Autodesk Fusion 360 part; units mm, degrees
note: some values were not read from the file. Set by a fixed rule: the direction of a hole.
(part 6 of 10)
  line L4790 (55.322, 32.9023) -> (55.808, 32.999)
  line L4791 (58.348, 32.999) -> (58.834, 32.9023)
  line L4792 (59.246, 32.627) -> (59.5213, 32.215)
  line L4793 (58.348, 30.459) -> (55.808, 30.459)
  line L4794 (55.808, 32.999) -> (58.348, 32.999)
  line L4795 (59.5213, 31.243) -> (59.246, 30.831)
  line L4796 (55.808, 30.459) -> (55.322, 30.5557)
  line L4797 (58.834, 32.9023) -> (59.246, 32.627)
  line L4798 (59.618, 31.729) -> (59.5213, 31.243)
  line L4799 (67.61, 55.627) -> (68.022, 55.9023)
  line L4800 (71.048, 55.999) -> (71.534, 55.9023)
  line L4801 (67.3347, 54.243) -> (67.238, 54.729)
  line L4802 (67.61, 53.831) -> (67.3347, 54.243)
  line L4803 (72.2213, 54.243) -> (71.946, 53.831)
  line L4804 (68.508, 53.459) -> (68.022, 53.5557)
  line L4805 (71.534, 53.5557) -> (71.048, 53.459)
  line L4806 (68.022, 53.5557) -> (67.61, 53.831)
  line L4807 (71.946, 53.831) -> (71.534, 53.5557)
  line L4808 (68.508, 55.999) -> (71.048, 55.999)
  line L4809 (72.2213, 55.215) -> (72.318, 54.729)
  line L4810 (68.022, 55.9023) -> (68.508, 55.999)
  line L4811 (71.946, 55.627) -> (72.2213, 55.215)
  line L4812 (71.048, 53.459) -> (68.508, 53.459)
  line L4813 (71.534, 55.9023) -> (71.946, 55.627)
  line L4814 (72.318, 54.729) -> (72.2213, 54.243)
  line L4815 (67.238, 54.729) -> (67.3347, 55.215)
  line L4816 (67.3347, 55.215) -> (67.61, 55.627)
  line L4817 (67.238, 31.729) -> (67.3347, 32.215)
  line L4818 (67.61, 30.831) -> (67.3347, 31.243)
  line L4819 (68.508, 30.459) -> (68.022, 30.5557)
  line L4820 (68.022, 30.5557) -> (67.61, 30.831)
  line L4821 (72.318, 31.729) -> (72.2213, 31.243)
  line L4822 (67.61, 32.627) -> (68.022, 32.9023)
  line L4823 (71.048, 32.999) -> (71.534, 32.9023)
  line L4824 (67.3347, 32.215) -> (67.61, 32.627)
  line L4825 (71.534, 30.5557) -> (71.048, 30.459)
  line L4826 (67.3347, 31.243) -> (67.238, 31.729)
  line L4827 (68.022, 32.9023) -> (68.508, 32.999)
  line L4828 (71.534, 32.9023) -> (71.946, 32.627)
  line L4829 (72.2213, 31.243) -> (71.946, 30.831)
  line L4830 (71.946, 32.627) -> (72.2213, 32.215)
  line L4831 (71.946, 30.831) -> (71.534, 30.5557)
  line L4832 (71.048, 30.459) -> (68.508, 30.459)
  line L4833 (72.2213, 32.215) -> (72.318, 31.729)
  line L4834 (68.508, 32.999) -> (71.048, 32.999)
  line L4835 (84.234, 55.9023) -> (84.646, 55.627)
  line L4836 (84.234, 53.5557) -> (83.748, 53.459)
  line L4837 (84.646, 55.627) -> (84.9213, 55.215)
  line L4838 (80.31, 53.831) -> (80.0347, 54.243)
  line L4839 (84.9213, 54.243) -> (84.646, 53.831)
  line L4840 (80.31, 55.627) -> (80.722, 55.9023)
  line L4841 (84.9213, 55.215) -> (85.018, 54.729)
  line L4842 (81.208, 53.459) -> (80.722, 53.5557)
  line L4843 (80.0347, 55.215) -> (80.31, 55.627)
  line L4844 (79.938, 54.729) -> (80.0347, 55.215)
  line L4845 (83.748, 53.459) -> (81.208, 53.459)
  line L4846 (80.722, 53.5557) -> (80.31, 53.831)
  line L4847 (85.018, 54.729) -> (84.9213, 54.243)
  line L4848 (81.208, 55.999) -> (83.748, 55.999)
  line L4849 (83.748, 55.999) -> (84.234, 55.9023)
  line L4850 (80.0347, 54.243) -> (79.938, 54.729)
  line L4851 (84.646, 53.831) -> (84.234, 53.5557)
  line L4852 (80.722, 55.9023) -> (81.208, 55.999)
  line L4853 (80.0347, 31.243) -> (79.938, 31.729)
  line L4854 (81.208, 32.999) -> (83.748, 32.999)
  line L4855 (80.722, 30.5557) -> (80.31, 30.831)
  line L4856 (84.646, 32.627) -> (84.9213, 32.215)
  line L4857 (80.31, 30.831) -> (80.0347, 31.243)
  line L4858 (84.9213, 32.215) -> (85.018, 31.729)
  line L4859 (80.0347, 32.215) -> (80.31, 32.627)
  line L4860 (84.234, 32.9023) -> (84.646, 32.627)
  line L4861 (83.748, 32.999) -> (84.234, 32.9023)
  line L4862 (84.646, 30.831) -> (84.234, 30.5557)
  line L4863 (81.208, 30.459) -> (80.722, 30.5557)
  line L4864 (83.748, 30.459) -> (81.208, 30.459)
  line L4865 (80.31, 32.627) -> (80.722, 32.9023)
  line L4866 (85.018, 31.729) -> (84.9213, 31.243)
  line L4867 (84.234, 30.5557) -> (83.748, 30.459)
  line L4868 (84.9213, 31.243) -> (84.646, 30.831)
  line L4869 (79.938, 31.729) -> (80.0347, 32.215)
  line L4870 (80.722, 32.9023) -> (81.208, 32.999)
  line L4871 (92.375, 55.627) -> (92.787, 55.9023)
  line L4872 (96.299, 55.9023) -> (96.711, 55.627)
  line L4873 (92.0997, 54.243) -> (92.003, 54.729)
  line L4874 (96.711, 55.627) -> (96.9863, 55.215)
  line L4875 (96.9863, 55.215) -> (97.083, 54.729)
  line L4876 (92.787, 55.9023) -> (93.273, 55.999)
  line L4877 (97.083, 54.729) -> (96.9863, 54.243)
  line L4878 (96.9863, 54.243) -> (96.711, 53.831)
  line L4879 (96.711, 53.831) -> (96.299, 53.5557)
  line L4880 (92.0997, 55.215) -> (92.375, 55.627)
  line L4881 (96.299, 53.5557) -> (95.813, 53.459)
  line L4882 (95.813, 55.999) -> (96.299, 55.9023)
  line L4883 (95.813, 53.459) -> (93.273, 53.459)
  line L4884 (93.273, 55.999) -> (95.813, 55.999)
  line L4885 (93.273, 53.459) -> (92.787, 53.5557)
  line L4886 (92.003, 54.729) -> (92.0997, 55.215)
  line L4887 (92.375, 53.831) -> (92.0997, 54.243)
  line L4888 (92.787, 53.5557) -> (92.375, 53.831)
  line L4889 (95.813, 30.459) -> (93.273, 30.459)
  line L4890 (92.0997, 32.215) -> (92.375, 32.627)
  line L4891 (92.003, 31.729) -> (92.0997, 32.215)
  line L4892 (95.813, 32.999) -> (96.299, 32.9023)
  line L4893 (96.9863, 31.243) -> (96.711, 30.831)
  line L4894 (92.0997, 31.243) -> (92.003, 31.729)
  line L4895 (93.273, 30.459) -> (92.787, 30.5557)
  line L4896 (92.787, 30.5557) -> (92.375, 30.831)
  line L4897 (93.273, 32.999) -> (95.813, 32.999)
  line L4898 (92.787, 32.9023) -> (93.273, 32.999)
  line L4899 (92.375, 32.627) -> (92.787, 32.9023)
  line L4900 (96.711, 32.627) -> (96.9863, 32.215)
  line L4901 (96.299, 32.9023) -> (96.711, 32.627)
  line L4902 (96.711, 30.831) -> (96.299, 30.5557)
  line L4903 (92.375, 30.831) -> (92.0997, 31.243)
  line L4904 (96.9863, 32.215) -> (97.083, 31.729)
  line L4905 (96.299, 30.5557) -> (95.813, 30.459)
  line L4906 (97.083, 31.729) -> (96.9863, 31.243)
  line L4907 (49.2301, 76.8268) -> (49.31, 76.425)
  line L4908 (47.8582, 77.3951) -> (48.26, 77.475)
  line L4909 (47.5175, 77.1675) -> (47.8582, 77.3951)
  line L4910 (48.26, 73.275) -> (47.8582, 73.3549)
  line L4911 (47.5175, 73.5825) -> (47.2899, 73.9232)
  line L4912 (48.6618, 73.3549) -> (48.26, 73.275)
  line L4913 (47.2899, 73.9232) -> (47.21, 74.325)
  line L4914 (49.0025, 73.5825) -> (48.6618, 73.3549)
  line L4915 (47.2899, 76.8268) -> (47.5175, 77.1675)
  line L4916 (49.0025, 77.1675) -> (49.2301, 76.8268)
  line L4917 (48.6618, 77.3951) -> (49.0025, 77.1675)
  line L4918 (48.26, 77.475) -> (48.6618, 77.3951)
  line L4919 (49.31, 76.425) -> (49.31, 74.325)
  line L4920 (47.8582, 73.3549) -> (47.5175, 73.5825)
  line L4921 (49.2301, 73.9232) -> (49.0025, 73.5825)
  line L4922 (47.21, 76.425) -> (47.2899, 76.8268)
  line L4923 (47.21, 74.325) -> (47.21, 76.425)
  line L4924 (49.31, 74.325) -> (49.2301, 73.9232)
  line L4925 (52.5975, 73.5825) -> (52.3699, 73.9232)
  line L4926 (54.39, 76.425) -> (54.39, 74.325)
  line L4927 (52.29, 76.425) -> (52.3699, 76.8268)
  line L4928 (52.3699, 76.8268) -> (52.5975, 77.1675)
  line L4929 (54.0825, 77.1675) -> (54.3101, 76.8268)
  line L4930 (52.29, 74.325) -> (52.29, 76.425)
  line L4931 (53.34, 77.475) -> (53.7418, 77.3951)
  line L4932 (54.39, 74.325) -> (54.3101, 73.9232)
  line L4933 (53.34, 73.275) -> (52.9382, 73.3549)
  line L4934 (54.3101, 76.8268) -> (54.39, 76.425)
  line L4935 (52.9382, 73.3549) -> (52.5975, 73.5825)
  line L4936 (54.0825, 73.5825) -> (53.7418, 73.3549)
  line L4937 (52.3699, 73.9232) -> (52.29, 74.325)
  line L4938 (53.7418, 77.3951) -> (54.0825, 77.1675)
  line L4939 (52.5975, 77.1675) -> (52.9382, 77.3951)
  line L4940 (52.9382, 77.3951) -> (53.34, 77.475)
  line L4941 (54.3101, 73.9232) -> (54.0825, 73.5825)
  line L4942 (53.7418, 73.3549) -> (53.34, 73.275)
  line L4943 (6.0868, 11.7651) -> (6.4275, 11.5375)
  line L4944 (6.4275, 11.5375) -> (6.6551, 11.1968)
  line L4945 (2.535, 10.795) -> (2.6149, 11.1968)
  line L4946 (6.6551, 11.1968) -> (6.735, 10.795)
  line L4947 (2.8425, 11.5375) -> (3.1832, 11.7651)
  line L4948 (2.6149, 11.1968) -> (2.8425, 11.5375)
  line L4949 (3.585, 9.745) -> (3.1832, 9.8249)
  line L4950 (6.735, 10.795) -> (6.6551, 10.3932)
  line L4951 (6.6551, 10.3932) -> (6.4275, 10.0525)
  line L4952 (5.685, 9.745) -> (3.585, 9.745)
  line L4953 (5.685, 11.845) -> (6.0868, 11.7651)
  line L4954 (3.1832, 11.7651) -> (3.585, 11.845)
  line L4955 (3.1832, 9.8249) -> (2.8425, 10.0525)
  line L4956 (2.6149, 10.3932) -> (2.535, 10.795)
  line L4957 (3.585, 11.845) -> (5.685, 11.845)
  line L4958 (6.0868, 9.8249) -> (5.685, 9.745)
  line L4959 (2.8425, 10.0525) -> (2.6149, 10.3932)
  line L4960 (6.4275, 10.0525) -> (6.0868, 9.8249)
  line L4961 (6.735, 15.875) -> (6.6551, 15.4732)
  line L4962 (6.0868, 16.8451) -> (6.4275, 16.6175)
  line L4963 (6.0868, 14.9049) -> (5.685, 14.825)
  line L4964 (2.8425, 16.6175) -> (3.1832, 16.8451)
  line L4965 (3.585, 16.925) -> (5.685, 16.925)
  line L4966 (6.4275, 16.6175) -> (6.6551, 16.2768)
  line L4967 (5.685, 14.825) -> (3.585, 14.825)
  line L4968 (3.1832, 16.8451) -> (3.585, 16.925)
  line L4969 (2.8425, 15.1325) -> (2.6149, 15.4732)
  line L4970 (6.6551, 15.4732) -> (6.4275, 15.1325)
  line L4971 (3.1832, 14.9049) -> (2.8425, 15.1325)
  line L4972 (2.535, 15.875) -> (2.6149, 16.2768)
  line L4973 (6.6551, 16.2768) -> (6.735, 15.875)
  line L4974 (6.4275, 15.1325) -> (6.0868, 14.9049)
  line L4975 (2.6149, 15.4732) -> (2.535, 15.875)
  line L4976 (5.685, 16.925) -> (6.0868, 16.8451)
  line L4977 (2.6149, 16.2768) -> (2.8425, 16.6175)
  line L4978 (3.585, 14.825) -> (3.1832, 14.9049)
  line L4979 (16.925, 5.94) -> (16.925, 3.84)
  line L4980 (16.6175, 3.0975) -> (16.2768, 2.8699)
  line L4981 (15.4732, 6.9101) -> (15.875, 6.99)
  line L4982 (15.4732, 2.8699) -> (15.1325, 3.0975)
  line L4983 (15.1325, 3.0975) -> (14.9049, 3.4382)
  line L4984 (16.8451, 6.3418) -> (16.925, 5.94)
  line L4985 (16.8451, 3.4382) -> (16.6175, 3.0975)
  line L4986 (15.875, 2.79) -> (15.4732, 2.8699)
  line L4987 (14.825, 3.84) -> (14.825, 5.94)
  line L4988 (16.2768, 6.9101) -> (16.6175, 6.6825)
  line L4989 (16.925, 3.84) -> (16.8451, 3.4382)
  line L4990 (15.1325, 6.6825) -> (15.4732, 6.9101)
  line L4991 (14.825, 5.94) -> (14.9049, 6.3418)
  line L4992 (16.2768, 2.8699) -> (15.875, 2.79)
  line L4993 (16.6175, 6.6825) -> (16.8451, 6.3418)
  line L4994 (15.875, 6.99) -> (16.2768, 6.9101)
  line L4995 (14.9049, 3.4382) -> (14.825, 3.84)
  line L4996 (14.9049, 6.3418) -> (15.1325, 6.6825)
  line L4997 (21.6975, 6.6825) -> (21.9251, 6.3418)
  line L4998 (20.955, 2.79) -> (20.5532, 2.8699)
  line L4999 (22.005, 3.84) -> (21.9251, 3.4382)
  line L5000 (20.5532, 2.8699) -> (20.2125, 3.0975)
  line L5001 (21.9251, 3.4382) -> (21.6975, 3.0975)
  line L5002 (20.955, 6.99) -> (21.3568, 6.9101)
  line L5003 (20.5532, 6.9101) -> (20.955, 6.99)
  line L5004 (19.905, 3.84) -> (19.905, 5.94)
  line L5005 (21.3568, 6.9101) -> (21.6975, 6.6825)
  line L5006 (22.005, 5.94) -> (22.005, 3.84)
  line L5007 (20.2125, 6.6825) -> (20.5532, 6.9101)
  line L5008 (19.905, 5.94) -> (19.9849, 6.3418)
  line L5009 (19.9849, 6.3418) -> (20.2125, 6.6825)
  line L5010 (21.9251, 6.3418) -> (22.005, 5.94)
  line L5011 (20.2125, 3.0975) -> (19.9849, 3.4382)
  line L5012 (19.9849, 3.4382) -> (19.905, 3.84)
  line L5013 (21.3568, 2.8699) -> (20.955, 2.79)
  line L5014 (21.6975, 3.0975) -> (21.3568, 2.8699)
  line L5015 (27.6049, 6.3418) -> (27.8325, 6.6825)
  line L5016 (27.525, 5.94) -> (27.6049, 6.3418)
  line L5017 (28.575, 2.79) -> (28.1732, 2.8699)
  line L5018 (29.5451, 6.3418) -> (29.625, 5.94)
  line L5019 (28.9768, 6.9101) -> (29.3175, 6.6825)
  line L5020 (27.525, 3.84) -> (27.525, 5.94)
  line L5021 (28.9768, 2.8699) -> (28.575, 2.79)
  line L5022 (29.625, 3.84) -> (29.5451, 3.4382)
  line L5023 (28.575, 6.99) -> (28.9768, 6.9101)
  line L5024 (27.8325, 6.6825) -> (28.1732, 6.9101)
  line L5025 (28.1732, 6.9101) -> (28.575, 6.99)
  line L5026 (29.625, 5.94) -> (29.625, 3.84)
  line L5027 (28.1732, 2.8699) -> (27.8325, 3.0975)
  line L5028 (29.3175, 3.0975) -> (28.9768, 2.8699)
  line L5029 (27.8325, 3.0975) -> (27.6049, 3.4382)
  line L5030 (29.3175, 6.6825) -> (29.5451, 6.3418)
  line L5031 (29.5451, 3.4382) -> (29.3175, 3.0975)
  line L5032 (27.6049, 3.4382) -> (27.525, 3.84)
  line L5033 (32.6849, 6.3418) -> (32.9125, 6.6825)
  line L5034 (33.655, 6.99) -> (34.0568, 6.9101)
  line L5035 (34.3975, 6.6825) -> (34.6251, 6.3418)
  line L5036 (34.0568, 6.9101) -> (34.3975, 6.6825)
  line L5037 (34.6251, 6.3418) -> (34.705, 5.94)
  line L5038 (34.705, 5.94) -> (34.705, 3.84)
  line L5039 (33.2532, 6.9101) -> (33.655, 6.99)
  line L5040 (33.655, 2.79) -> (33.2532, 2.8699)
  line L5041 (32.605, 3.84) -> (32.605, 5.94)
  line L5042 (33.2532, 2.8699) -> (32.9125, 3.0975)
  line L5043 (32.9125, 6.6825) -> (33.2532, 6.9101)
  line L5044 (34.6251, 3.4382) -> (34.3975, 3.0975)
  line L5045 (34.0568, 2.8699) -> (33.655, 2.79)
  line L5046 (34.3975, 3.0975) -> (34.0568, 2.8699)
  line L5047 (32.6849, 3.4382) -> (32.605, 3.84)
  line L5048 (32.9125, 3.0975) -> (32.6849, 3.4382)
  line L5049 (34.705, 3.84) -> (34.6251, 3.4382)
  line L5050 (32.605, 5.94) -> (32.6849, 6.3418)
  line L5051 (40.5325, 6.6825) -> (40.8732, 6.9101)
  line L5052 (40.8732, 2.8699) -> (40.5325, 3.0975)
  line L5053 (42.2451, 3.4382) -> (42.0175, 3.0975)
  line L5054 (40.3049, 3.4382) -> (40.225, 3.84)
  line L5055 (40.5325, 3.0975) -> (40.3049, 3.4382)
  line L5056 (41.275, 6.99) -> (41.6768, 6.9101)
  line L5057 (41.6768, 2.8699) -> (41.275, 2.79)
  line L5058 (40.3049, 6.3418) -> (40.5325, 6.6825)
  line L5059 (40.225, 3.84) -> (40.225, 5.94)
  line L5060 (40.8732, 6.9101) -> (41.275, 6.99)
  line L5061 (40.225, 5.94) -> (40.3049, 6.3418)
  line L5062 (42.325, 5.94) -> (42.325, 3.84)
  line L5063 (42.0175, 6.6825) -> (42.2451, 6.3418)
  line L5064 (42.0175, 3.0975) -> (41.6768, 2.8699)
  line L5065 (41.6768, 6.9101) -> (42.0175, 6.6825)
  line L5066 (42.2451, 6.3418) -> (42.325, 5.94)
  line L5067 (41.275, 2.79) -> (40.8732, 2.8699)
  line L5068 (42.325, 3.84) -> (42.2451, 3.4382)
  line L5069 (46.355, 6.99) -> (46.7568, 6.9101)
  line L5070 (47.0975, 3.0975) -> (46.7568, 2.8699)
  line L5071 (47.405, 5.94) -> (47.405, 3.84)
  line L5072 (45.9532, 2.8699) -> (45.6125, 3.0975)
  line L5073 (45.3849, 3.4382) -> (45.305, 3.84)
  line L5074 (45.9532, 6.9101) -> (46.355, 6.99)
  line L5075 (45.6125, 6.6825) -> (45.9532, 6.9101)
  line L5076 (45.305, 5.94) -> (45.3849, 6.3418)
  line L5077 (47.405, 3.84) -> (47.3251, 3.4382)
  line L5078 (45.305, 3.84) -> (45.305, 5.94)
  line L5079 (46.7568, 2.8699) -> (46.355, 2.79)
  line L5080 (46.7568, 6.9101) -> (47.0975, 6.6825)
  line L5081 (47.3251, 3.4382) -> (47.0975, 3.0975)
  line L5082 (45.6125, 3.0975) -> (45.3849, 3.4382)
  line L5083 (46.355, 2.79) -> (45.9532, 2.8699)
  line L5084 (45.3849, 6.3418) -> (45.6125, 6.6825)
  line L5085 (47.0975, 6.6825) -> (47.3251, 6.3418)
  line L5086 (47.3251, 6.3418) -> (47.405, 5.94)
  line L5087 (55.5801, 3.4382) -> (55.3525, 3.0975)
  line L5088 (55.3525, 3.0975) -> (55.0118, 2.8699)
  line L5089 (54.2082, 6.9101) -> (54.61, 6.99)
  line L5090 (55.0118, 6.9101) -> (55.3525, 6.6825)
  line L5091 (55.3525, 6.6825) -> (55.5801, 6.3418)
  line L5092 (53.6399, 6.3418) -> (53.8675, 6.6825)
  line L5093 (55.5801, 6.3418) -> (55.66, 5.94)
  line L5094 (55.66, 5.94) -> (55.66, 3.84)
  line L5095 (54.61, 2.79) -> (54.2082, 2.8699)
  line L5096 (53.8675, 3.0975) -> (53.6399, 3.4382)
  line L5097 (54.61, 6.99) -> (55.0118, 6.9101)
  line L5098 (55.0118, 2.8699) -> (54.61, 2.79)
  line L5099 (53.6399, 3.4382) -> (53.56, 3.84)
  line L5100 (55.66, 3.84) -> (55.5801, 3.4382)
  line L5101 (53.56, 5.94) -> (53.6399, 6.3418)
  line L5102 (53.8675, 6.6825) -> (54.2082, 6.9101)
  line L5103 (53.56, 3.84) -> (53.56, 5.94)
  line L5104 (54.2082, 2.8699) -> (53.8675, 3.0975)
  line L5105 (58.64, 5.94) -> (58.7199, 6.3418)
  line L5106 (60.4325, 3.0975) -> (60.0918, 2.8699)
  line L5107 (59.2882, 2.8699) -> (58.9475, 3.0975)
  line L5108 (60.74, 3.84) -> (60.6601, 3.4382)
  line L5109 (60.0918, 2.8699) -> (59.69, 2.79)
  line L5110 (59.69, 2.79) -> (59.2882, 2.8699)
  line L5111 (58.64, 3.84) -> (58.64, 5.94)
  line L5112 (60.4325, 6.6825) -> (60.6601, 6.3418)
  line L5113 (60.6601, 3.4382) -> (60.4325, 3.0975)
  line L5114 (58.9475, 3.0975) -> (58.7199, 3.4382)
  line L5115 (58.7199, 3.4382) -> (58.64, 3.84)
  line L5116 (60.6601, 6.3418) -> (60.74, 5.94)
  line L5117 (60.74, 5.94) -> (60.74, 3.84)
  line L5118 (58.7199, 6.3418) -> (58.9475, 6.6825)
  line L5119 (59.69, 6.99) -> (60.0918, 6.9101)
  line L5120 (60.0918, 6.9101) -> (60.4325, 6.6825)
  line L5121 (59.2882, 6.9101) -> (59.69, 6.99)
  line L5122 (58.9475, 6.6825) -> (59.2882, 6.9101)
  line L5123 (67.31, 2.79) -> (66.9082, 2.8699)
  line L5124 (68.0525, 6.6825) -> (68.2801, 6.3418)
  line L5125 (66.26, 5.94) -> (66.3399, 6.3418)
  line L5126 (66.9082, 2.8699) -> (66.5675, 3.0975)
  line L5127 (68.36, 3.84) -> (68.2801, 3.4382)
  line L5128 (66.3399, 3.4382) -> (66.26, 3.84)
  line L5129 (66.9082, 6.9101) -> (67.31, 6.99)
  line L5130 (68.2801, 6.3418) -> (68.36, 5.94)
  line L5131 (66.3399, 6.3418) -> (66.5675, 6.6825)
  line L5132 (67.31, 6.99) -> (67.7118, 6.9101)
  line L5133 (67.7118, 2.8699) -> (67.31, 2.79)
  line L5134 (66.5675, 3.0975) -> (66.3399, 3.4382)
  line L5135 (68.2801, 3.4382) -> (68.0525, 3.0975)
  line L5136 (66.26, 3.84) -> (66.26, 5.94)
  line L5137 (68.36, 5.94) -> (68.36, 3.84)
  line L5138 (68.0525, 3.0975) -> (67.7118, 2.8699)
  line L5139 (66.5675, 6.6825) -> (66.9082, 6.9101)
  line L5140 (67.7118, 6.9101) -> (68.0525, 6.6825)
  line L5141 (73.44, 5.94) -> (73.44, 3.84)
  line L5142 (73.3601, 6.3418) -> (73.44, 5.94)
  line L5143 (71.34, 5.94) -> (71.4199, 6.3418)
  line L5144 (71.6475, 6.6825) -> (71.9882, 6.9101)
  line L5145 (71.9882, 2.8699) -> (71.6475, 3.0975)
  line L5146 (72.7918, 6.9101) -> (73.1325, 6.6825)
  line L5147 (72.39, 2.79) -> (71.9882, 2.8699)
  line L5148 (72.39, 6.99) -> (72.7918, 6.9101)
  line L5149 (73.44, 3.84) -> (73.3601, 3.4382)
  line L5150 (71.4199, 3.4382) -> (71.34, 3.84)
  line L5151 (71.4199, 6.3418) -> (71.6475, 6.6825)
  line L5152 (73.1325, 6.6825) -> (73.3601, 6.3418)
  line L5153 (73.1325, 3.0975) -> (72.7918, 2.8699)
  line L5154 (72.7918, 2.8699) -> (72.39, 2.79)
  line L5155 (71.34, 3.84) -> (71.34, 5.94)
  line L5156 (71.9882, 6.9101) -> (72.39, 6.99)
  line L5157 (71.6475, 3.0975) -> (71.4199, 3.4382)
  line L5158 (73.3601, 3.4382) -> (73.1325, 3.0975)
  line L5159 (80.01, 2.79) -> (79.6082, 2.8699)
  line L5160 (80.4118, 2.8699) -> (80.01, 2.79)
  line L5161 (80.7525, 3.0975) -> (80.4118, 2.8699)
  line L5162 (80.9801, 6.3418) -> (81.06, 5.94)
  line L5163 (79.6082, 6.9101) -> (80.01, 6.99)
  line L5164 (79.0399, 6.3418) -> (79.2675, 6.6825)
  line L5165 (79.2675, 3.0975) -> (79.0399, 3.4382)
  line L5166 (79.0399, 3.4382) -> (78.96, 3.84)
  line L5167 (80.9801, 3.4382) -> (80.7525, 3.0975)
  line L5168 (79.6082, 2.8699) -> (79.2675, 3.0975)
  line L5169 (79.2675, 6.6825) -> (79.6082, 6.9101)
  line L5170 (78.96, 3.84) -> (78.96, 5.94)
  line L5171 (80.4118, 6.9101) -> (80.7525, 6.6825)
  line L5172 (80.7525, 6.6825) -> (80.9801, 6.3418)
  line L5173 (81.06, 3.84) -> (80.9801, 3.4382)
  line L5174 (80.01, 6.99) -> (80.4118, 6.9101)
  line L5175 (78.96, 5.94) -> (79.0399, 6.3418)
  line L5176 (81.06, 5.94) -> (81.06, 3.84)
  line L5177 (84.1199, 3.4382) -> (84.04, 3.84)
  line L5178 (85.09, 2.79) -> (84.6882, 2.8699)
  line L5179 (84.04, 5.94) -> (84.1199, 6.3418)
  line L5180 (86.0601, 6.3418) -> (86.14, 5.94)
  line L5181 (85.8325, 6.6825) -> (86.0601, 6.3418)
  line L5182 (85.8325, 3.0975) -> (85.4918, 2.8699)
  line L5183 (84.6882, 2.8699) -> (84.3475, 3.0975)
  line L5184 (84.6882, 6.9101) -> (85.09, 6.99)
  line L5185 (84.3475, 3.0975) -> (84.1199, 3.4382)
  line L5186 (86.14, 3.84) -> (86.0601, 3.4382)
  line L5187 (84.04, 3.84) -> (84.04, 5.94)
  line L5188 (86.0601, 3.4382) -> (85.8325, 3.0975)
  line L5189 (84.1199, 6.3418) -> (84.3475, 6.6825)
  line L5190 (86.14, 5.94) -> (86.14, 3.84)
  line L5191 (85.4918, 2.8699) -> (85.09, 2.79)
  line L5192 (85.09, 6.99) -> (85.4918, 6.9101)
  line L5193 (84.3475, 6.6825) -> (84.6882, 6.9101)
  line L5194 (85.4918, 6.9101) -> (85.8325, 6.6825)
  line L5195 (96.49, 11.845) -> (96.8918, 11.7651)
  line L5196 (93.6475, 11.5375) -> (93.9882, 11.7651)
  line L5197 (97.54, 10.795) -> (97.4601, 10.3932)
  line L5198 (94.39, 11.845) -> (96.49, 11.845)
  line L5199 (93.6475, 10.0525) -> (93.4199, 10.3932)
  line L5200 (97.2325, 11.5375) -> (97.4601, 11.1968)
  line L5201 (93.34, 10.795) -> (93.4199, 11.1968)
  line L5202 (94.39, 9.745) -> (93.9882, 9.8249)
  line L5203 (96.8918, 11.7651) -> (97.2325, 11.5375)
  line L5204 (93.9882, 11.7651) -> (94.39, 11.845)
  line L5205 (96.49, 9.745) -> (94.39, 9.745)
  line L5206 (97.4601, 11.1968) -> (97.54, 10.795)
  line L5207 (97.2325, 10.0525) -> (96.8918, 9.8249)
  line L5208 (97.4601, 10.3932) -> (97.2325, 10.0525)
  line L5209 (93.9882, 9.8249) -> (93.6475, 10.0525)
  line L5210 (93.4199, 11.1968) -> (93.6475, 11.5375)
  line L5211 (93.4199, 10.3932) -> (93.34, 10.795)
  line L5212 (96.8918, 9.8249) -> (96.49, 9.745)
  line L5213 (93.4199, 16.2768) -> (93.6475, 16.6175)
  line L5214 (93.9882, 16.8451) -> (94.39, 16.925)
  line L5215 (94.39, 14.825) -> (93.9882, 14.9049)
  line L5216 (97.4601, 15.4732) -> (97.2325, 15.1325)
  line L5217 (93.9882, 14.9049) -> (93.6475, 15.1325)
  line L5218 (96.49, 14.825) -> (94.39, 14.825)
  line L5219 (96.49, 16.925) -> (96.8918, 16.8451)
  line L5220 (96.8918, 14.9049) -> (96.49, 14.825)
  line L5221 (97.4601, 16.2768) -> (97.54, 15.875)
  line L5222 (97.54, 15.875) -> (97.4601, 15.4732)
  line L5223 (93.6475, 16.6175) -> (93.9882, 16.8451)
  line L5224 (97.2325, 16.6175) -> (97.4601, 16.2768)
  line L5225 (96.8918, 16.8451) -> (97.2325, 16.6175)
  line L5226 (93.6475, 15.1325) -> (93.4199, 15.4732)
  line L5227 (97.2325, 15.1325) -> (96.8918, 14.9049)
  line L5228 (93.34, 15.875) -> (93.4199, 16.2768)
  line L5229 (94.39, 16.925) -> (96.49, 16.925)
  line L5230 (93.4199, 15.4732) -> (93.34, 15.875)
  line L5231 (22.2504, 77.1652) -> (22.2504, 76.5048)
  line L5232 (21.2598, 77.4954) -> (21.9202, 77.4954)
  line L5233 (21.9202, 77.4954) -> (22.2504, 77.1652)
  line L5234 (21.2598, 76.1746) -> (20.9296, 76.5048)
  line L5235 (20.9296, 77.1652) -> (21.2598, 77.4954)
  line L5236 (20.9296, 76.5048) -> (20.9296, 77.1652)
  line L5237 (21.9202, 76.1746) -> (21.2598, 76.1746)
  line L5238 (22.2504, 76.5048) -> (21.9202, 76.1746)
  line L5239 (23.7998, 76.1746) -> (23.4696, 76.5048)
  line L5240 (24.7904, 77.1652) -> (24.7904, 76.5048)
  line L5241 (24.4602, 77.4954) -> (24.7904, 77.1652)
  line L5242 (24.7904, 76.5048) -> (24.4602, 76.1746)
  line L5243 (24.4602, 76.1746) -> (23.7998, 76.1746)
  line L5244 (23.7998, 77.4954) -> (24.4602, 77.4954)
  line L5245 (23.4696, 76.5048) -> (23.4696, 77.1652)
  line L5246 (23.4696, 77.1652) -> (23.7998, 77.4954)
  line L5247 (78.4098, 75.5396) -> (78.0796, 75.8698)
  line L5248 (78.4098, 76.8604) -> (79.0702, 76.8604)
  line L5249 (78.0796, 76.5302) -> (78.4098, 76.8604)
  line L5250 (79.0702, 75.5396) -> (78.4098, 75.5396)
  line L5251 (79.4004, 76.5302) -> (79.4004, 75.8698)
  line L5252 (79.4004, 75.8698) -> (79.0702, 75.5396)
  line L5253 (78.0796, 75.8698) -> (78.0796, 76.5302)
  line L5254 (79.0702, 76.8604) -> (79.4004, 76.5302)
  line L5255 (75.8698, 75.5396) -> (75.5396, 75.8698)
  line L5256 (76.5302, 75.5396) -> (75.8698, 75.5396)
  line L5257 (76.8604, 76.5302) -> (76.8604, 75.8698)
  line L5258 (75.5396, 76.5302) -> (75.8698, 76.8604)
  line L5259 (76.8604, 75.8698) -> (76.5302, 75.5396)
  line L5260 (76.5302, 76.8604) -> (76.8604, 76.5302)
  line L5261 (75.5396, 75.8698) -> (75.5396, 76.5302)
  line L5262 (75.8698, 76.8604) -> (76.5302, 76.8604)
  line L5263 (10.8204, 16.8402) -> (10.8204, 16.1798)
  line L5264 (10.8204, 16.1798) -> (10.4902, 15.8496)
  line L5265 (9.4996, 16.1798) -> (9.4996, 16.8402)
  line L5266 (10.4902, 17.1704) -> (10.8204, 16.8402)
  line L5267 (9.8298, 17.1704) -> (10.4902, 17.1704)
  line L5268 (10.4902, 15.8496) -> (9.8298, 15.8496)
  line L5269 (9.8298, 15.8496) -> (9.4996, 16.1798)
  line L5270 (9.4996, 16.8402) -> (9.8298, 17.1704)
  line L5271 (12.0396, 16.8402) -> (12.3698, 17.1704)
  line L5272 (13.0302, 15.8496) -> (12.3698, 15.8496)
  line L5273 (13.0302, 17.1704) -> (13.3604, 16.8402)
  line L5274 (12.3698, 15.8496) -> (12.0396, 16.1798)
  line L5275 (12.3698, 17.1704) -> (13.0302, 17.1704)
  line L5276 (13.3604, 16.8402) -> (13.3604, 16.1798)
  line L5277 (12.0396, 16.1798) -> (12.0396, 16.8402)
  line L5278 (13.3604, 16.1798) -> (13.0302, 15.8496)
  line L5279 (79.4004, 16.8402) -> (79.4004, 16.1798)
  line L5280 (78.0796, 16.1798) -> (78.0796, 16.8402)
  line L5281 (79.4004, 16.1798) -> (79.0702, 15.8496)
  line L5282 (78.0796, 16.8402) -> (78.4098, 17.1704)
  line L5283 (79.0702, 15.8496) -> (78.4098, 15.8496)
  line L5284 (79.0702, 17.1704) -> (79.4004, 16.8402)
  line L5285 (78.4098, 17.1704) -> (79.0702, 17.1704)
  line L5286 (78.4098, 15.8496) -> (78.0796, 16.1798)
  line L5287 (75.8698, 17.1704) -> (76.5302, 17.1704)
  line L5288 (76.8604, 16.1798) -> (76.5302, 15.8496)
  line L5289 (76.8604, 16.8402) -> (76.8604, 16.1798)
  line L5290 (76.5302, 17.1704) -> (76.8604, 16.8402)
  line L5291 (75.8698, 15.8496) -> (75.5396, 16.1798)
  line L5292 (75.5396, 16.8402) -> (75.8698, 17.1704)
  line L5293 (75.5396, 16.1798) -> (75.5396, 16.8402)
  line L5294 (76.5302, 15.8496) -> (75.8698, 15.8496)
  line L5295 (66.9798, 17.1704) -> (67.6402, 17.1704)
  line L5296 (67.6402, 17.1704) -> (67.9704, 16.8402)
  line L5297 (66.9798, 15.8496) -> (66.6496, 16.1798)
  line L5298 (66.6496, 16.1798) -> (66.6496, 16.8402)
  line L5299 (67.9704, 16.8402) -> (67.9704, 16.1798)
  line L5300 (67.9704, 16.1798) -> (67.6402, 15.8496)
  line L5301 (66.6496, 16.8402) -> (66.9798, 17.1704)
  line L5302 (67.6402, 15.8496) -> (66.9798, 15.8496)
  line L5303 (64.4398, 15.8496) -> (64.1096, 16.1798)
  line L5304 (64.4398, 17.1704) -> (65.1002, 17.1704)
  line L5305 (64.1096, 16.1798) -> (64.1096, 16.8402)
  line L5306 (65.1002, 15.8496) -> (64.4398, 15.8496)
  line L5307 (64.1096, 16.8402) -> (64.4398, 17.1704)
  line L5308 (65.1002, 17.1704) -> (65.4304, 16.8402)
  line L5309 (65.4304, 16.1798) -> (65.1002, 15.8496)
  line L5310 (65.4304, 16.8402) -> (65.4304, 16.1798)
  line L5311 (57.8104, 16.1798) -> (57.4802, 15.8496)
  line L5312 (56.8198, 15.8496) -> (56.4896, 16.1798)
  line L5313 (56.8198, 17.1704) -> (57.4802, 17.1704)
  line L5314 (57.4802, 15.8496) -> (56.8198, 15.8496)
  line L5315 (56.4896, 16.1798) -> (56.4896, 16.8402)
  line L5316 (57.8104, 16.8402) -> (57.8104, 16.1798)
  line L5317 (56.4896, 16.8402) -> (56.8198, 17.1704)
  line L5318 (57.4802, 17.1704) -> (57.8104, 16.8402)
  line L5319 (54.2798, 15.8496) -> (53.9496, 16.1798)
  line L5320 (54.2798, 17.1704) -> (54.9402, 17.1704)
  line L5321 (55.2704, 16.8402) -> (55.2704, 16.1798)
  line L5322 (54.9402, 15.8496) -> (54.2798, 15.8496)
  line L5323 (55.2704, 16.1798) -> (54.9402, 15.8496)
  line L5324 (54.9402, 17.1704) -> (55.2704, 16.8402)
  line L5325 (53.9496, 16.8402) -> (54.2798, 17.1704)
  line L5326 (53.9496, 16.1798) -> (53.9496, 16.8402)
  line L5327 (46.0248, 17.1704) -> (46.6852, 17.1704)
  line L5328 (46.6852, 17.1704) -> (47.0154, 16.8402)
  line L5329 (47.0154, 16.8402) -> (47.0154, 16.1798)
  line L5330 (45.6946, 16.1798) -> (45.6946, 16.8402)
  line L5331 (45.6946, 16.8402) -> (46.0248, 17.1704)
  line L5332 (46.6852, 15.8496) -> (46.0248, 15.8496)
  line L5333 (46.0248, 15.8496) -> (45.6946, 16.1798)
  line L5334 (47.0154, 16.1798) -> (46.6852, 15.8496)
  line L5335 (48.5648, 17.1704) -> (49.2252, 17.1704)
  line L5336 (49.5554, 16.1798) -> (49.2252, 15.8496)
  line L5337 (48.5648, 15.8496) -> (48.2346, 16.1798)
  line L5338 (49.2252, 17.1704) -> (49.5554, 16.8402)
  line L5339 (48.2346, 16.1798) -> (48.2346, 16.8402)
  line L5340 (48.2346, 16.8402) -> (48.5648, 17.1704)
  line L5341 (49.2252, 15.8496) -> (48.5648, 15.8496)
  line L5342 (49.5554, 16.8402) -> (49.5554, 16.1798)
  line L5343 (36.2204, 16.8402) -> (36.2204, 16.1798)
  line L5344 (35.2298, 15.8496) -> (34.8996, 16.1798)
  line L5345 (34.8996, 16.8402) -> (35.2298, 17.1704)
  line L5346 (35.8902, 15.8496) -> (35.2298, 15.8496)
  line L5347 (36.2204, 16.1798) -> (35.8902, 15.8496)
  line L5348 (34.8996, 16.1798) -> (34.8996, 16.8402)
  line L5349 (35.2298, 17.1704) -> (35.8902, 17.1704)
  line L5350 (35.8902, 17.1704) -> (36.2204, 16.8402)
  line L5351 (38.4302, 17.1704) -> (38.7604, 16.8402)
  line L5352 (38.7604, 16.1798) -> (38.4302, 15.8496)
  line L5353 (37.4396, 16.8402) -> (37.7698, 17.1704)
  line L5354 (38.4302, 15.8496) -> (37.7698, 15.8496)
  line L5355 (38.7604, 16.8402) -> (38.7604, 16.1798)
  line L5356 (37.7698, 17.1704) -> (38.4302, 17.1704)
  line L5357 (37.7698, 15.8496) -> (37.4396, 16.1798)
  line L5358 (37.4396, 16.1798) -> (37.4396, 16.8402)
  line L5359 (22.1996, 16.8402) -> (22.5298, 17.1704)
  line L5360 (22.5298, 17.1704) -> (23.1902, 17.1704)
  line L5361 (23.1902, 15.8496) -> (22.5298, 15.8496)
  line L5362 (22.5298, 15.8496) -> (22.1996, 16.1798)
  line L5363 (23.5204, 16.8402) -> (23.5204, 16.1798)
  line L5364 (23.5204, 16.1798) -> (23.1902, 15.8496)
  line L5365 (22.1996, 16.1798) -> (22.1996, 16.8402)
  line L5366 (23.1902, 17.1704) -> (23.5204, 16.8402)
  line L5367 (25.7302, 15.8496) -> (25.0698, 15.8496)
  line L5368 (24.7396, 16.1798) -> (24.7396, 16.8402)
  line L5369 (24.7396, 16.8402) -> (25.0698, 17.1704)
  line L5370 (26.0604, 16.8402) -> (26.0604, 16.1798)
  line L5371 (26.0604, 16.1798) -> (25.7302, 15.8496)
  line L5372 (25.0698, 17.1704) -> (25.7302, 17.1704)
  line L5373 (25.0698, 15.8496) -> (24.7396, 16.1798)
  line L5374 (25.7302, 17.1704) -> (26.0604, 16.8402)
  line L5375 (89.5096, 16.1798) -> (89.5096, 16.8402)
  line L5376 (90.5002, 15.8496) -> (89.8398, 15.8496)
  line L5377 (89.8398, 15.8496) -> (89.5096, 16.1798)
  line L5378 (90.8304, 16.8402) -> (90.8304, 16.1798)
  line L5379 (90.5002, 17.1704) -> (90.8304, 16.8402)
  line L5380 (89.5096, 16.8402) -> (89.8398, 17.1704)
  line L5381 (89.8398, 17.1704) -> (90.5002, 17.1704)
  line L5382 (90.8304, 16.1798) -> (90.5002, 15.8496)
  line L5383 (86.9696, 16.8402) -> (87.2998, 17.1704)
  line L5384 (86.9696, 16.1798) -> (86.9696, 16.8402)
  line L5385 (88.2904, 16.1798) -> (87.9602, 15.8496)
  line L5386 (87.9602, 15.8496) -> (87.2998, 15.8496)
  line L5387 (87.2998, 17.1704) -> (87.9602, 17.1704)
  line L5388 (87.9602, 17.1704) -> (88.2904, 16.8402)
  line L5389 (87.2998, 15.8496) -> (86.9696, 16.1798)
  line L5390 (88.2904, 16.8402) -> (88.2904, 16.1798)
  line L5391 (19.3802, 77.4954) -> (19.7104, 77.1652)
  line L5392 (19.7104, 76.5048) -> (19.3802, 76.1746)
  line L5393 (18.3896, 76.5048) -> (18.3896, 77.1652)
  line L5394 (19.3802, 76.1746) -> (18.7198, 76.1746)
  line L5395 (19.7104, 77.1652) -> (19.7104, 76.5048)
  line L5396 (18.7198, 76.1746) -> (18.3896, 76.5048)
  line L5397 (18.7198, 77.4954) -> (19.3802, 77.4954)
  line L5398 (18.3896, 77.1652) -> (18.7198, 77.4954)
  line L5399 (9.2202, 77.4954) -> (9.5504, 77.1652)
  line L5400 (8.5598, 77.4954) -> (9.2202, 77.4954)
  line L5401 (8.2296, 77.1652) -> (8.5598, 77.4954)
  line L5402 (9.2202, 76.1746) -> (8.5598, 76.1746)
  line L5403 (8.2296, 76.5048) -> (8.2296, 77.1652)
  line L5404 (8.5598, 76.1746) -> (8.2296, 76.5048)
  line L5405 (9.5504, 76.5048) -> (9.2202, 76.1746)
  line L5406 (9.5504, 77.1652) -> (9.5504, 76.5048)
  line L5407 (80.9498, 76.8604) -> (81.6102, 76.8604)
  line L5408 (80.6196, 75.8698) -> (80.6196, 76.5302)
  line L5409 (80.9498, 75.5396) -> (80.6196, 75.8698)
  line L5410 (81.6102, 76.8604) -> (81.9404, 76.5302)
  line L5411 (81.9404, 76.5302) -> (81.9404, 75.8698)
  line L5412 (81.6102, 75.5396) -> (80.9498, 75.5396)
  line L5413 (81.9404, 75.8698) -> (81.6102, 75.5396)
  line L5414 (80.6196, 76.5302) -> (80.9498, 76.8604)
  line L5415 (90.7796, 75.8698) -> (90.7796, 76.5302)
  line L5416 (91.1098, 75.5396) -> (90.7796, 75.8698)
  line L5417 (91.7702, 75.5396) -> (91.1098, 75.5396)
  line L5418 (92.1004, 75.8698) -> (91.7702, 75.5396)
  line L5419 (91.1098, 76.8604) -> (91.7702, 76.8604)
  line L5420 (92.1004, 76.5302) -> (92.1004, 75.8698)
  line L5421 (91.7702, 76.8604) -> (92.1004, 76.5302)
  line L5422 (90.7796, 76.5302) -> (91.1098, 76.8604)
  line L5423 (9.8298, 20.9804) -> (10.4902, 20.9804)
  line L5424 (10.8204, 20.6502) -> (10.8204, 19.9898)
  line L5425 (9.4996, 20.6502) -> (9.8298, 20.9804)
  line L5426 (10.4902, 20.9804) -> (10.8204, 20.6502)
  line L5427 (9.8298, 19.6596) -> (9.4996, 19.9898)
  line L5428 (10.4902, 19.6596) -> (9.8298, 19.6596)
  line L5429 (9.4996, 19.9898) -> (9.4996, 20.6502)
  line L5430 (10.8204, 19.9898) -> (10.4902, 19.6596)
  line L5431 (10.8204, 30.8102) -> (10.8204, 30.1498)
  line L5432 (10.4902, 29.8196) -> (9.8298, 29.8196)
  line L5433 (9.8298, 29.8196) -> (9.4996, 30.1498)
  line L5434 (9.4996, 30.8102) -> (9.8298, 31.1404)
  line L5435 (10.4902, 31.1404) -> (10.8204, 30.8102)
  line L5436 (9.4996, 30.1498) -> (9.4996, 30.8102)
  line L5437 (10.8204, 30.1498) -> (10.4902, 29.8196)
  line L5438 (9.8298, 31.1404) -> (10.4902, 31.1404)
  line L5439 (22.5298, 19.6596) -> (22.1996, 19.9898)
  line L5440 (22.1996, 20.6502) -> (22.5298, 20.9804)
  line L5441 (22.5298, 20.9804) -> (23.1902, 20.9804)
  line L5442 (22.1996, 19.9898) -> (22.1996, 20.6502)
  line L5443 (23.5204, 20.6502) -> (23.5204, 19.9898)
  line L5444 (23.1902, 19.6596) -> (22.5298, 19.6596)
  line L5445 (23.1902, 20.9804) -> (23.5204, 20.6502)
  line L5446 (23.5204, 19.9898) -> (23.1902, 19.6596)
  line L5447 (23.5204, 30.1498) -> (23.1902, 29.8196)
  line L5448 (22.1996, 30.8102) -> (22.5298, 31.1404)
  line L5449 (23.5204, 30.8102) -> (23.5204, 30.1498)
  line L5450 (23.1902, 29.8196) -> (22.5298, 29.8196)
  line L5451 (22.1996, 30.1498) -> (22.1996, 30.8102)
  line L5452 (22.5298, 31.1404) -> (23.1902, 31.1404)
  line L5453 (22.5298, 29.8196) -> (22.1996, 30.1498)
  line L5454 (23.1902, 31.1404) -> (23.5204, 30.8102)
  line L5455 (35.8902, 20.9804) -> (36.2204, 20.6502)
  line L5456 (36.2204, 19.9898) -> (35.8902, 19.6596)
  line L5457 (36.2204, 20.6502) -> (36.2204, 19.9898)
  line L5458 (35.2298, 19.6596) -> (34.8996, 19.9898)
  line L5459 (34.8996, 20.6502) -> (35.2298, 20.9804)
  line L5460 (34.8996, 19.9898) -> (34.8996, 20.6502)
  line L5461 (35.8902, 19.6596) -> (35.2298, 19.6596)
  line L5462 (35.2298, 20.9804) -> (35.8902, 20.9804)
  line L5463 (34.8996, 30.1498) -> (34.8996, 30.8102)
  line L5464 (34.8996, 30.8102) -> (35.2298, 31.1404)
  line L5465 (36.2204, 30.1498) -> (35.8902, 29.8196)
  line L5466 (35.2298, 29.8196) -> (34.8996, 30.1498)
  line L5467 (35.8902, 31.1404) -> (36.2204, 30.8102)
  line L5468 (36.2204, 30.8102) -> (36.2204, 30.1498)
  line L5469 (35.8902, 29.8196) -> (35.2298, 29.8196)
  line L5470 (35.2298, 31.1404) -> (35.8902, 31.1404)
  line L5471 (47.5996, 20.6502) -> (47.9298, 20.9804)
  line L5472 (48.9204, 20.6502) -> (48.9204, 19.9898)
  line L5473 (48.5902, 20.9804) -> (48.9204, 20.6502)
  line L5474 (47.9298, 19.6596) -> (47.5996, 19.9898)
  line L5475 (47.5996, 19.9898) -> (47.5996, 20.6502)
  line L5476 (47.9298, 20.9804) -> (48.5902, 20.9804)
  line L5477 (48.9204, 19.9898) -> (48.5902, 19.6596)
  line L5478 (48.5902, 19.6596) -> (47.9298, 19.6596)
  line L5479 (47.5996, 30.1498) -> (47.5996, 30.8102)
  line L5480 (48.5902, 31.1404) -> (48.9204, 30.8102)
  line L5481 (47.9298, 29.8196) -> (47.5996, 30.1498)
  line L5482 (47.9298, 31.1404) -> (48.5902, 31.1404)
  line L5483 (47.5996, 30.8102) -> (47.9298, 31.1404)
  line L5484 (48.9204, 30.8102) -> (48.9204, 30.1498)
  line L5485 (48.5902, 29.8196) -> (47.9298, 29.8196)
  line L5486 (48.9204, 30.1498) -> (48.5902, 29.8196)
  line L5487 (54.0004, 19.9898) -> (53.6702, 19.6596)
  line L5488 (52.6796, 19.9898) -> (52.6796, 20.6502)
  line L5489 (53.6702, 20.9804) -> (54.0004, 20.6502)
  line L5490 (53.0098, 20.9804) -> (53.6702, 20.9804)
  line L5491 (52.6796, 20.6502) -> (53.0098, 20.9804)
  line L5492 (53.0098, 19.6596) -> (52.6796, 19.9898)
  line L5493 (53.6702, 19.6596) -> (53.0098, 19.6596)
  line L5494 (54.0004, 20.6502) -> (54.0004, 19.9898)
  line L5495 (54.0004, 30.8102) -> (54.0004, 30.1498)
  line L5496 (53.0098, 31.1404) -> (53.6702, 31.1404)
  line L5497 (52.6796, 30.8102) -> (53.0098, 31.1404)
  line L5498 (53.6702, 31.1404) -> (54.0004, 30.8102)
  line L5499 (53.6702, 29.8196) -> (53.0098, 29.8196)
  line L5500 (53.0098, 29.8196) -> (52.6796, 30.1498)
  line L5501 (54.0004, 30.1498) -> (53.6702, 29.8196)
  line L5502 (52.6796, 30.1498) -> (52.6796, 30.8102)
  line L5503 (66.6496, 20.6502) -> (66.9798, 20.9804)
  line L5504 (67.9704, 20.6502) -> (67.9704, 19.9898)
  line L5505 (67.6402, 20.9804) -> (67.9704, 20.6502)
  line L5506 (67.9704, 19.9898) -> (67.6402, 19.6596)
  line L5507 (66.9798, 20.9804) -> (67.6402, 20.9804)
  line L5508 (66.9798, 19.6596) -> (66.6496, 19.9898)
  line L5509 (66.6496, 19.9898) -> (66.6496, 20.6502)
  line L5510 (67.6402, 19.6596) -> (66.9798, 19.6596)
  line L5511 (66.6496, 30.1498) -> (66.6496, 30.8102)
  line L5512 (66.9798, 31.1404) -> (67.6402, 31.1404)
  line L5513 (66.6496, 30.8102) -> (66.9798, 31.1404)
  line L5514 (66.9798, 29.8196) -> (66.6496, 30.1498)
  line L5515 (67.6402, 29.8196) -> (66.9798, 29.8196)
  line L5516 (67.6402, 31.1404) -> (67.9704, 30.8102)
  line L5517 (67.9704, 30.8102) -> (67.9704, 30.1498)
  line L5518 (67.9704, 30.1498) -> (67.6402, 29.8196)
  line L5519 (79.0702, 20.9804) -> (79.4004, 20.6502)
  line L5520 (78.0796, 20.6502) -> (78.4098, 20.9804)
  line L5521 (78.4098, 19.6596) -> (78.0796, 19.9898)
  line L5522 (78.0796, 19.9898) -> (78.0796, 20.6502)
  line L5523 (79.4004, 20.6502) -> (79.4004, 19.9898)
  line L5524 (79.4004, 19.9898) -> (79.0702, 19.6596)
  line L5525 (79.0702, 19.6596) -> (78.4098, 19.6596)
  line L5526 (78.4098, 20.9804) -> (79.0702, 20.9804)
  line L5527 (78.4098, 29.8196) -> (78.0796, 30.1498)
  line L5528 (78.0796, 30.8102) -> (78.4098, 31.1404)
  line L5529 (78.0796, 30.1498) -> (78.0796, 30.8102)
  line L5530 (79.0702, 31.1404) -> (79.4004, 30.8102)
  line L5531 (79.0702, 29.8196) -> (78.4098, 29.8196)
  line L5532 (79.4004, 30.1498) -> (79.0702, 29.8196)
  line L5533 (78.4098, 31.1404) -> (79.0702, 31.1404)
  line L5534 (79.4004, 30.8102) -> (79.4004, 30.1498)
  line L5535 (89.5096, 19.9898) -> (89.5096, 20.6502)
  line L5536 (89.8398, 20.9804) -> (90.5002, 20.9804)
  line L5537 (90.8304, 20.6502) -> (90.8304, 19.9898)
  line L5538 (89.5096, 20.6502) -> (89.8398, 20.9804)
  line L5539 (90.8304, 19.9898) -> (90.5002, 19.6596)
  line L5540 (90.5002, 19.6596) -> (89.8398, 19.6596)
  line L5541 (90.5002, 20.9804) -> (90.8304, 20.6502)
  line L5542 (89.8398, 19.6596) -> (89.5096, 19.9898)
  line L5543 (90.8304, 30.1498) -> (90.5002, 29.8196)
  line L5544 (90.8304, 30.8102) -> (90.8304, 30.1498)
  line L5545 (90.5002, 31.1404) -> (90.8304, 30.8102)
  line L5546 (89.5096, 30.1498) -> (89.5096, 30.8102)
  line L5547 (89.8398, 31.1404) -> (90.5002, 31.1404)
  line L5548 (89.8398, 29.8196) -> (89.5096, 30.1498)
  line L5549 (89.5096, 30.8102) -> (89.8398, 31.1404)
  line L5550 (90.5002, 29.8196) -> (89.8398, 29.8196)
  line L5551 (34.2565, 77.2996) -> (34.7234, 77.7666)
  line L5552 (35.6574, 76.8326) -> (35.1904, 76.3657)
  line L5553 (34.7234, 77.7666) -> (35.1904, 77.7666)
  line L5554 (34.2565, 76.8326) -> (34.2565, 77.2996)
  line L5555 (35.1904, 76.3657) -> (34.7234, 76.3657)
  line L5556 (35.6574, 77.2996) -> (35.6574, 76.8326)
  line L5557 (34.7234, 76.3657) -> (34.2565, 76.8326)
  line L5558 (35.1904, 77.7666) -> (35.6574, 77.2996)
  line L5559 (42.3746, 69.1815) -> (41.9076, 69.1815)
  line L5560 (42.8416, 69.6484) -> (42.3746, 69.1815)
  line L5561 (42.8416, 70.1154) -> (42.8416, 69.6484)
  line L5562 (41.4407, 70.1154) -> (41.9076, 70.5824)
  line L5563 (42.3746, 70.5824) -> (42.8416, 70.1154)
  line L5564 (41.9076, 69.1815) -> (41.4407, 69.6484)
  line L5565 (41.9076, 70.5824) -> (42.3746, 70.5824)
  line L5566 (41.4407, 69.6484) -> (41.4407, 70.1154)
  line L5567 (29.5402, 77.4954) -> (29.8704, 77.1652)
  line L5568 (29.5402, 76.1746) -> (28.8798, 76.1746)
  line L5569 (28.8798, 76.1746) -> (28.5496, 76.5048)
  line L5570 (29.8704, 77.1652) -> (29.8704, 76.5048)
  line L5571 (28.5496, 76.5048) -> (28.5496, 77.1652)
  line L5572 (29.8704, 76.5048) -> (29.5402, 76.1746)
  line L5573 (28.8798, 77.4954) -> (29.5402, 77.4954)
  line L5574 (28.5496, 77.1652) -> (28.8798, 77.4954)
  line L5575 (26.3398, 76.1746) -> (26.0096, 76.5048)
  line L5576 (27.0002, 76.1746) -> (26.3398, 76.1746)
  line L5577 (27.3304, 77.1652) -> (27.3304, 76.5048)
  line L5578 (27.0002, 77.4954) -> (27.3304, 77.1652)
  line L5579 (26.0096, 77.1652) -> (26.3398, 77.4954)
  line L5580 (26.3398, 77.4954) -> (27.0002, 77.4954)
  line L5581 (27.3304, 76.5048) -> (27.0002, 76.1746)
  line L5582 (26.0096, 76.5048) -> (26.0096, 77.1652)
  line L5583 (10.795, 76.5302) -> (10.795, 77.1398)
  line L5584 (9.9314, 77.1398) -> (9.9314, 76.5302)
  line L5585 (9.9314, 76.5302) -> (10.795, 76.5302)
  line L5586 (10.795, 77.1398) -> (9.9314, 77.1398)
  line L5587 (18.0086, 77.1398) -> (17.145, 77.1398)
  line L5588 (17.145, 77.1398) -> (17.145, 76.5302)
  line L5589 (18.0086, 76.5302) -> (18.0086, 77.1398)
  line L5590 (17.145, 76.5302) -> (18.0086, 76.5302)
  line L5591 (89.535, 75.8952) -> (90.3986, 75.8952)
  line L5592 (89.535, 76.5048) -> (89.535, 75.8952)
  line L5593 (90.3986, 75.8952) -> (90.3986, 76.5048)
  line L5594 (90.3986, 76.5048) -> (89.535, 76.5048)
  line L5595 (83.185, 75.8952) -> (83.185, 76.5048)
  line L5596 (83.185, 76.5048) -> (82.3214, 76.5048)
  line L5597 (82.3214, 76.5048) -> (82.3214, 75.8952)
  line L5598 (82.3214, 75.8952) -> (83.185, 75.8952)
  line L5599 (10.4648, 29.4386) -> (9.8552, 29.4386)
  line L5600 (9.8552, 29.4386) -> (9.8552, 28.575)
  line L5601 (10.4648, 28.575) -> (10.4648, 29.4386)
  line L5602 (9.8552, 28.575) -> (10.4648, 28.575)
  line L5603 (9.8552, 21.3614) -> (10.4648, 21.3614)
  line L5604 (10.4648, 22.225) -> (9.8552, 22.225)
  line L5605 (9.8552, 22.225) -> (9.8552, 21.3614)
  line L5606 (10.4648, 21.3614) -> (10.4648, 22.225)
  line L5607 (22.5552, 28.575) -> (23.1648, 28.575)
  line L5608 (22.5552, 29.4386) -> (22.5552, 28.575)
  line L5609 (23.1648, 29.4386) -> (22.5552, 29.4386)
  line L5610 (23.1648, 28.575) -> (23.1648, 29.4386)
  line L5611 (22.5552, 21.3614) -> (23.1648, 21.3614)
  line L5612 (23.1648, 22.225) -> (22.5552, 22.225)
  line L5613 (22.5552, 22.225) -> (22.5552, 21.3614)
  line L5614 (23.1648, 21.3614) -> (23.1648, 22.225)
  line L5615 (35.2552, 28.575) -> (35.8648, 28.575)
  line L5616 (35.2552, 29.4386) -> (35.2552, 28.575)
  line L5617 (35.8648, 29.4386) -> (35.2552, 29.4386)
  line L5618 (35.8648, 28.575) -> (35.8648, 29.4386)
  line L5619 (35.2552, 21.3614) -> (35.8648, 21.3614)
  line L5620 (35.8648, 22.225) -> (35.2552, 22.225)
  line L5621 (35.2552, 22.225) -> (35.2552, 21.3614)
  line L5622 (35.8648, 21.3614) -> (35.8648, 22.225)
  line L5623 (48.5648, 28.575) -> (48.5648, 29.4386)
  line L5624 (48.5648, 29.4386) -> (47.9552, 29.4386)
  line L5625 (47.9552, 29.4386) -> (47.9552, 28.575)
  line L5626 (47.9552, 28.575) -> (48.5648, 28.575)
  line L5627 (47.9552, 22.225) -> (47.9552, 21.3614)
  line L5628 (48.5648, 21.3614) -> (48.5648, 22.225)
  line L5629 (47.9552, 21.3614) -> (48.5648, 21.3614)
  line L5630 (48.5648, 22.225) -> (47.9552, 22.225)
  line L5631 (53.6448, 29.4386) -> (53.0352, 29.4386)
  line L5632 (53.0352, 28.575) -> (53.6448, 28.575)
  line L5633 (53.6448, 28.575) -> (53.6448, 29.4386)
  line L5634 (53.0352, 29.4386) -> (53.0352, 28.575)
  line L5635 (53.6448, 21.3614) -> (53.6448, 22.225)
  line L5636 (53.6448, 22.225) -> (53.0352, 22.225)
  line L5637 (53.0352, 22.225) -> (53.0352, 21.3614)
  line L5638 (53.0352, 21.3614) -> (53.6448, 21.3614)
  line L5639 (67.0052, 29.4386) -> (67.0052, 28.575)
  line L5640 (67.6148, 28.575) -> (67.6148, 29.4386)
  line L5641 (67.6148, 29.4386) -> (67.0052, 29.4386)
  line L5642 (67.0052, 28.575) -> (67.6148, 28.575)
  line L5643 (67.0052, 22.225) -> (67.0052, 21.3614)
  line L5644 (67.6148, 21.3614) -> (67.6148, 22.225)
  line L5645 (67.6148, 22.225) -> (67.0052, 22.225)
  line L5646 (67.0052, 21.3614) -> (67.6148, 21.3614)
  line L5647 (79.0448, 29.4386) -> (78.4352, 29.4386)
  line L5648 (78.4352, 28.575) -> (79.0448, 28.575)
  line L5649 (78.4352, 29.4386) -> (78.4352, 28.575)
  line L5650 (79.0448, 28.575) -> (79.0448, 29.4386)
  line L5651 (79.0448, 21.3614) -> (79.0448, 22.225)
  line L5652 (79.0448, 22.225) -> (78.4352, 22.225)
  line L5653 (78.4352, 22.225) -> (78.4352, 21.3614)
  line L5654 (78.4352, 21.3614) -> (79.0448, 21.3614)
  line L5655 (89.8652, 28.575) -> (90.4748, 28.575)
  line L5656 (90.4748, 29.4386) -> (89.8652, 29.4386)
  line L5657 (89.8652, 29.4386) -> (89.8652, 28.575)
  line L5658 (90.4748, 28.575) -> (90.4748, 29.4386)
  line L5659 (90.4748, 22.225) -> (89.8652, 22.225)
  line L5660 (89.8652, 21.3614) -> (90.4748, 21.3614)
  line L5661 (89.8652, 22.225) -> (89.8652, 21.3614)
  line L5662 (90.4748, 21.3614) -> (90.4748, 22.225)
  line L5663 (41.1892, 70.4028) -> (41.6203, 70.8338)
  line L5664 (40.5786, 71.0134) -> (41.1892, 70.4028)
  line L5665 (41.0096, 71.4445) -> (40.5786, 71.0134)
  line L5666 (41.6203, 70.8338) -> (41.0096, 71.4445)
  line L5667 (35.9088, 76.5453) -> (35.4778, 76.1142)
  line L5668 (36.0884, 75.5036) -> (36.5195, 75.9346)
  line L5669 (36.5195, 75.9346) -> (35.9088, 76.5453)
  line L5670 (35.4778, 76.1142) -> (36.0884, 75.5036)
  arc A0 (21.77, 64.695) -> (18.77, 64.695) centre (20.27, 64.695) ccw
  arc A1 (18.77, 64.695) -> (21.77, 64.695) centre (20.27, 64.695) ccw
  arc A2 (81.56, 64.845) -> (78.56, 64.845) centre (80.06, 64.845) ccw
  arc A3 (78.56, 64.845) -> (81.56, 64.845) centre (80.06, 64.845) ccw
  arc A4 (4.143, 43.229) -> (7.143, 43.229) centre (5.643, 43.229) ccw
  arc A5 (7.143, 43.229) -> (4.143, 43.229) centre (5.643, 43.229) ccw
  arc A6 (16.843, 43.229) -> (19.843, 43.229) centre (18.343, 43.229) ccw
  arc A7 (19.843, 43.229) -> (16.843, 43.229) centre (18.343, 43.229) ccw
  arc A8 (29.543, 43.229) -> (32.543, 43.229) centre (31.043, 43.229) ccw
  arc A9 (32.543, 43.229) -> (29.543, 43.229) centre (31.043, 43.229) ccw
  arc A10 (45.243, 43.229) -> (42.243, 43.229) centre (43.743, 43.229) ccw
  arc A11 (42.243, 43.229) -> (45.243, 43.229) centre (43.743, 43.229) ccw
  arc A12 (58.578, 43.229) -> (55.578, 43.229) centre (57.078, 43.229) ccw
  arc A13 (55.578, 43.229) -> (58.578, 43.229) centre (57.078, 43.229) ccw
  arc A14 (71.278, 43.229) -> (68.278, 43.229) centre (69.778, 43.229) ccw
  arc A15 (68.278, 43.229) -> (71.278, 43.229) centre (69.778, 43.229) ccw
  arc A16 (80.978, 43.229) -> (83.978, 43.229) centre (82.478, 43.229) ccw
  arc A17 (83.978, 43.229) -> (80.978, 43.229) centre (82.478, 43.229) ccw
  arc A18 (96.043, 43.229) -> (93.043, 43.229) centre (94.543, 43.229) ccw
  arc A19 (93.043, 43.229) -> (96.043, 43.229) centre (94.543, 43.229) ccw
  arc A20 (46.66, 75.375) -> (49.86, 75.375) centre (48.26, 75.375) ccw
  arc A21 (49.86, 75.375) -> (46.66, 75.375) centre (48.26, 75.375) ccw
  arc A22 (54.94, 75.375) -> (51.74, 75.375) centre (53.34, 75.375) ccw
  arc A23 (51.74, 75.375) -> (54.94, 75.375) centre (53.34, 75.375) ccw
  arc A24 (6.235, 10.795) -> (3.035, 10.795) centre (4.635, 10.795) ccw
  arc A25 (3.035, 10.795) -> (6.235, 10.795) centre (4.635, 10.795) ccw
  line L5671 (6.235, 10.795) -> (6.235, 10.795)
  line L5672 (6.235, 15.875) -> (6.235, 15.875)
  arc A26 (3.035, 15.875) -> (6.235, 15.875) centre (4.635, 15.875) ccw
  arc A27 (6.235, 15.875) -> (3.035, 15.875) centre (4.635, 15.875) ccw
  arc A28 (17.475, 4.89) -> (14.275, 4.89) centre (15.875, 4.89) ccw
  arc A29 (14.275, 4.89) -> (17.475, 4.89) centre (15.875, 4.89) ccw
  line L5673 (22.555, 4.89) -> (22.555, 4.89)
  arc A30 (19.355, 4.89) -> (22.555, 4.89) centre (20.955, 4.89) ccw
  arc A31 (22.555, 4.89) -> (19.355, 4.89) centre (20.955, 4.89) ccw
  arc A32 (30.175, 4.89) -> (26.975, 4.89) centre (28.575, 4.89) ccw
  line L5674 (30.175, 4.89) -> (30.175, 4.89)
  arc A33 (26.975, 4.89) -> (30.175, 4.89) centre (28.575, 4.89) ccw
  arc A34 (35.255, 4.89) -> (32.055, 4.89) centre (33.655, 4.89) ccw
  arc A35 (32.055, 4.89) -> (35.255, 4.89) centre (33.655, 4.89) ccw
  arc A36 (42.875, 4.89) -> (39.675, 4.89) centre (41.275, 4.89) ccw
  arc A37 (39.675, 4.89) -> (42.875, 4.89) centre (41.275, 4.89) ccw
  arc A38 (47.955, 4.89) -> (44.755, 4.89) centre (46.355, 4.89) ccw
  arc A39 (44.755, 4.89) -> (47.955, 4.89) centre (46.355, 4.89) ccw
  arc A40 (53.01, 4.89) -> (56.21, 4.89) centre (54.61, 4.89) ccw
  arc A41 (56.21, 4.89) -> (53.01, 4.89) centre (54.61, 4.89) ccw
  arc A42 (58.09, 4.89) -> (61.29, 4.89) centre (59.69, 4.89) ccw
  arc A43 (61.29, 4.89) -> (58.09, 4.89) centre (59.69, 4.89) ccw
  arc A44 (68.91, 4.89) -> (65.71, 4.89) centre (67.31, 4.89) ccw
  arc A45 (65.71, 4.89) -> (68.91, 4.89) centre (67.31, 4.89) ccw
  arc A46 (70.79, 4.89) -> (73.99, 4.89) centre (72.39, 4.89) ccw
  arc A47 (73.99, 4.89) -> (70.79, 4.89) centre (72.39, 4.89) ccw
  arc A48 (81.61, 4.89) -> (78.41, 4.89) centre (80.01, 4.89) ccw
  arc A49 (78.41, 4.89) -> (81.61, 4.89) centre (80.01, 4.89) ccw
  arc A50 (86.69, 4.89) -> (83.49, 4.89) centre (85.09, 4.89) ccw
  arc A51 (83.49, 4.89) -> (86.69, 4.89) centre (85.09, 4.89) ccw
  arc A52 (97.04, 10.795) -> (93.84, 10.795) centre (95.44, 10.795) ccw